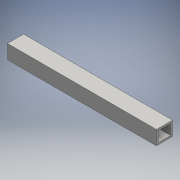
# Autodesk Inventor part: caja perfil
Saved by Autodesk Inventor 2016 (Build 200138000, 138)
## iProperties
Created: 2016-06-24
Part Number: caja perfil
Material: Generic
Document SubType Name: Modeling
Designer: Admin
Density: 1 g/cm^3
Appearance: Default
Author: Admin
Autodesk Inventor part; units mm, degrees
ref_plane "YZ Plane" through (0, 0, 0) normal (1, 0, 0) x (0, 1, 0)
ref_plane "XZ Plane" through (0, 0, 0) normal (0, 1, 0) x (-1, 0, 0)
ref_plane "XY Plane" through (0, 0, 0) normal (0, 0, 1) x (1, 0, 0)
sketch "Sketch2" plane through (0, 0, 0) normal (1, 0, 0) x (0, 1, 0)
  line L0 (0, 0) -> (17, 0)
  line L1 (17, 0) -> (17, -15)
  line L2 (17, -15) -> (0, -15)
  line L3 (0, -15) -> (0, 0)
  dimension "d4" = 17
  dimension "d5" = 15
  constraints: 8 end point, 2 parallel, 1 horizontal, 1 perpendicular
  measures "d4" distance of L1.end L2.end
  measures "d5" distance of L0.end L1.end
extrude "Extrusion2" add sketch "Sketch2" along normal blind 157
sketch "Sketch3" plane through (157, 0, 0) normal (1, 0, 0) x (0, 0, -1)
  line L0 (0, 17) -> (0, 0) projected
  line L1 (0, 0) -> (15, 0) projected
  line L2 (15, 0) -> (15, 17) projected
  line L3 (2, 2) -> (13, 2)
  line L4 (13, 2) -> (13, 15)
  line L5 (13, 15) -> (2, 15)
  line L6 (2, 15) -> (2, 2)
  line L7 (2, 2) -> (13, 15) construction
  line L8 (13, 2) -> (2, 15) construction
  point P0 (7.5, 8.5)
  dimension "d9" = 11
  dimension "d10" = 13
  constraints: 12 end point, 2 midpoint, 2 parallel, 1 horizontal, 1 perpendicular
  measures "d9" distance of L3.start L3.end
  measures "d10" distance of L4.end L3.end
extrude "Extrusion3" cut sketch "Sketch3" against normal through all
body "Solid2"
